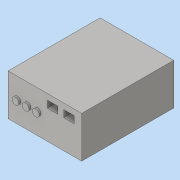
# Autodesk Inventor part: WR_LEN
Saved by Autodesk Inventor 2016 (Build 200138000, 138)
## iProperties
Created: 2016-09-19
Part Number: WR_LEN
Material: Generic
Document SubType Name: Modeling
Designer: Zara
Density: 1 g/cm^3
Appearance: Default
Voltage: 5.000 V
Current: 1.600 A
Power: 8.000 W
Author: Zara
Autodesk Inventor part; units mm, degrees
ref_plane "YZ Plane" through (0, 0, 0) normal (1, 0, 0) x (0, 1, 0)
ref_plane "XZ Plane" through (0, 0, 0) normal (0, 1, 0) x (-1, 0, 0)
ref_plane "XY Plane" through (0, 0, 0) normal (0, 0, 1) x (1, 0, 0)
sketch "Sketch1" plane through (0, 0, 0) normal (0, 0, 1) x (1, 0, 0)
  line L0 (-50.8, -28.575) -> (50.8, -28.575)
  line L1 (50.8, -28.575) -> (50.8, 28.575)
  line L2 (50.8, 28.575) -> (-50.8, 28.575)
  line L3 (-50.8, 28.575) -> (-50.8, -28.575)
  line L4 (-50.8, -28.575) -> (50.8, 28.575) construction
  line L5 (50.8, -28.575) -> (-50.8, 28.575) construction
  point P0 (0, 0)
  dimension "d0" = 101.6
  dimension "d1" = 57.15
  constraints: 12 end point, 2 midpoint, 2 parallel, 1 horizontal, 1 perpendicular
  measures "d0" distance of L1.end L2.end
  measures "d1" distance of L0.end L1.end
extrude "WR-LEN" add sketch "Sketch1" against normal blind 127
sketch "Sketch2" plane through (0, 0, 0) normal (0, 0, 1) x (1, 0, 0)
  line L0 (3.5309, 20.7371) -> (17.8184, 20.7371)
  line L1 (17.8184, 20.7371) -> (17.8184, 11.2121)
  line L2 (17.8184, 11.2121) -> (3.5309, 11.2121)
  line L3 (3.5309, 11.2121) -> (3.5309, 20.7371)
  line L4 (3.5309, 20.7371) -> (17.8184, 11.2121) construction
  line L5 (17.8184, 20.7371) -> (3.5309, 11.2121) construction
  line L6 (26.1201, 20.7371) -> (40.4265, 20.7371)
  line L7 (40.4265, 20.7371) -> (40.4265, 11.2121)
  line L8 (40.4265, 11.2121) -> (26.1201, 11.2121)
  line L9 (26.1201, 11.2121) -> (26.1201, 20.7371)
  point P0 (0, 0)
  point P1 (10.6746, 15.9746)
  dimension "d4" = 9.525
  dimension "d5" = 14.2875
  constraints: 20 end point, 4 parallel, 2 horizontal, 2 midpoint, 2 perpendicular
  measures "d4" distance of L0.end L1.end
  measures "d5" distance of L0.start L0.end
extrude "sfp ports" cut sketch "Sketch2" against normal blind 12.7
sketch "Sketch3" plane through (0, 0, 0) normal (0, 0, 1) x (1, 0, 0)
  circle A0 centre (-38.1, 0) radius 4.8133
  line L0 (-50.8, 28.575) -> (-50.8, -28.575) projected
  line L1 (50.8, 28.575) -> (-50.8, 28.575) projected
  circle A1 centre (-24.13, 0) radius 4.8133
  circle A2 centre (-10.16, 0) radius 4.8133
  point P0 (0, 0)
  dimension "d9" = 9.6266
  dimension "d10" = 12.7
  dimension "d11" = 28.575
  dimension "d14" = 13.97
  constraints: 3 centre point, 1 horizontal, 4 other
  measures "d9" diameter of A0
  measures "d10" distance from line of A0.centre L0
  measures "d11" distance from line of L1 A0.centre
  measures "d14" distance of A0.centre A1.centre
extrude "Extrusion3" add sketch "Sketch3" along normal blind 2.54
body "Solid1"
